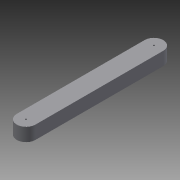
# Autodesk Inventor part: Conveyor Belt
Saved by Autodesk Inventor 2015 (Build 190159000, 159)
## iProperties
Created: 2014-10-18
Part Number: Conveyor Belt
Material: Generic
Document SubType Name: Modeling
Designer: jesse
Density: 1 g/cm^3
Appearance: Default
Author: jesse
Autodesk Inventor part; units mm, degrees
ref_plane "YZ Plane" through (0, 0, 0) normal (1, 0, 0) x (0, 1, 0)
ref_plane "XZ Plane" through (0, 0, 0) normal (0, 1, 0) x (-1, 0, 0)
ref_plane "XY Plane" through (0, 0, 0) normal (0, 0, 1) x (1, 0, 0)
sketch "Sketch1" plane through (0, 0, 0) normal (0, 1, 0) x (-1, 0, 0)
  arc A0 (60.868, 230.9741) -> (5.369, 230.9741) centre (33.1185, 230.9741) ccw
  arc A1 (5.369, -150.0259) -> (60.868, -150.0259) centre (33.1185, -150.0259) ccw
  line L0 (60.868, 230.9741) -> (60.868, -150.0259)
  line L1 (5.369, -150.0259) -> (5.369, 230.9741)
  line L2 (33.1185, -150.0259) -> (-189.304, -150.0259) construction
  line L3 (33.1185, 230.9741) -> (-194.5746, 230.9741) construction
  point P0 (0, 0)
  dimension "d0" = 55.499
  dimension "d1" = 381
  constraints: 8 end point, 4 point on circle, 4 tangent, 2 centre point, 2 horizontal, 2 point on line, 1 equal radius, 1 vertical
  measures "d0" diameter of A0
  measures "d1" distance between parallel lines of L2 L3
extrude "Extrusion1" add sketch "Sketch1" along normal blind 39.497
sketch "Sketch2" plane through (0, 39.497, 0) normal (0, 1, 0) x (1, 0, 0)
  arc A0 (-60.868, -230.9741) -> (-5.369, -230.9741) centre (-33.1185, -230.9741) ccw projected
  line L0 (-5.369, -230.9741) -> (-5.369, 150.0259) projected
  arc A1 (-5.369, 150.0259) -> (-60.868, 150.0259) centre (-33.1185, 150.0259) ccw projected
  line L1 (-60.868, 150.0259) -> (-60.868, -230.9741) projected
  circle A2 centre (-33.1185, -230.9741) radius 2.3495
  circle A3 centre (-33.1185, 150.0259) radius 2.3495
  point P0 (0, 0)
  dimension "d4" = 4.699
  dimension "d5" = 4.699
  constraints: 2 centre point, 2 coincident
  measures "d4" diameter of A2
  measures "d5" diameter of A3
extrude "Extrusion2" cut sketch "Sketch2" against normal through all contours A2 | A3
body "Solid1"
